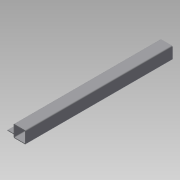
# Autodesk Inventor part: 9005
Saved by Autodesk Inventor 2013 (Build 170138000, 138)
## iProperties
Created: 2014-04-23
Part Number: 9005
Material: Generic
Document SubType Name: Modeling
Density: 1 g/cm^3
Vendor: 80/20 Inc.
Engineer: Ross Bowman
Designer: Ross Bowman
Catalog Web Link: 8020.net
Company: 80/20 Inc.
Author: Ross Bowman
Keywords: 80/20 , 8020 , T-Slot , Extrusion
Material: 6105-T5 Aluminum
Autodesk Inventor part; units mm, degrees
ref_plane "YZ Plane" through (0, 0, 0) normal (1, 0, 0) x (0, 1, 0)
ref_plane "XZ Plane" through (0, 0, 0) normal (0, 1, 0) x (-1, 0, 0)
ref_plane "XY Plane" through (0, 0, 0) normal (0, 0, 1) x (1, 0, 0)
sketch "Sketch1" plane through (0, 0, 0) normal (0, 0, 1) x (1, 0, 0)
  arc A0 (9.652, -11.176) -> (11.176, -9.652) centre (9.652, -9.652) ccw
  line L0 (-9.652, -11.176) -> (9.652, -11.176)
  arc A1 (-11.176, -9.652) -> (-9.652, -11.176) centre (-9.652, -9.652) ccw
  line L1 (-11.176, 9.652) -> (-11.176, -9.652)
  arc A2 (-9.652, 11.176) -> (-11.176, 9.652) centre (-9.652, 9.652) ccw
  line L2 (9.652, 11.176) -> (-9.652, 11.176)
  arc A3 (11.176, 9.652) -> (9.652, 11.176) centre (9.652, 9.652) ccw
  line L3 (11.176, -9.652) -> (11.176, 9.652)
  arc A4 (-12.7, -7.112) -> (-13.462, -6.35) centre (-13.462, -7.112) ccw
  line L4 (-12.7, -7.112) -> (-12.7, -10.5918)
  arc A5 (-12.7, -10.5918) -> (-10.5918, -12.7) centre (-10.5918, -10.5918) ccw
  line L5 (-10.5918, -12.7) -> (10.5918, -12.7)
  arc A6 (10.5918, -12.7) -> (12.7, -10.5918) centre (10.5918, -10.5918) ccw
  line L6 (12.7, -10.5918) -> (12.7, 10.5918)
  arc A7 (12.7, 10.5918) -> (10.5918, 12.7) centre (10.5918, 10.5918) ccw
  line L7 (10.5918, 12.7) -> (-10.5918, 12.7)
  arc A8 (-10.5918, 12.7) -> (-12.7, 10.5918) centre (-10.5918, 10.5918) ccw
  line L8 (-12.7, 10.5918) -> (-12.7, -4.064)
  arc A9 (-13.462, -4.826) -> (-12.7, -4.064) centre (-13.462, -4.064) ccw
  line L9 (-13.462, -4.826) -> (-24.638, -4.826)
  arc A10 (-24.638, -4.826) -> (-24.638, -6.35) centre (-24.638, -5.588) ccw
  line L10 (-24.638, -6.35) -> (-13.462, -6.35)
  point P0 (0, 0)
  constraints: 22 end point, 22 point on circle, 22 tangent, 11 centre point, 8 parallel, 1 collinear, 1 horizontal, 1 vertical
extrude "Extrusion1" add sketch "Sketch1" against normal blind 304.8
body "Solid1"
